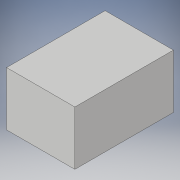
# Autodesk Inventor part: Part1
Saved by Autodesk Inventor 2019 (Build 230136000, 136)
## iProperties
Created: 2020-10-29
Part Number: Part1
Material: 一般
Document SubType Name: Modeling
Designer: kmol2020
Density: 1 g/cm^3
Appearance: 預設
Author: kmol2020
Autodesk Inventor part; units mm, degrees
ref_plane "YZ Plane" through (0, 0, 0) normal (1, 0, 0) x (0, 1, 0)
ref_plane "XZ Plane" through (0, 0, 0) normal (0, 1, 0) x (-1, 0, 0)
ref_plane "XY Plane" through (0, 0, 0) normal (0, 0, 1) x (1, 0, 0)
sketch "草圖1" plane through (0, 0, 0) normal (0, 1, 0) x (-1, 0, 0)
  line L0 (7.4046, 15.0148) -> (-5.2449, 15.0148)
  line L1 (-5.2449, 15.0148) -> (-5.2449, -3.2395)
  line L2 (-5.2449, -3.2395) -> (7.4046, -3.2395)
  line L3 (7.4046, -3.2395) -> (7.4046, 15.0148)
  point P0 (0, 0)
  dimension "d0" = 18.2543
  dimension "d1" = 12.6495
  constraints: 8 end point, 2 parallel, 1 horizontal, 1 perpendicular
  measures "d0" distance of L2.end L0.start
  measures "d1" distance of L1.end L2.end
extrude "擠出1" add sketch "草圖1" along normal blind 10
